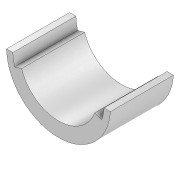
# Autodesk Inventor part: Back cover of tilting head
Saved by Autodesk Inventor 2020.3 (Build 243373010, 373A)
## iProperties
Created: 2021-05-15
Part Number: Back cover of tilting head
Material: Stainless Steel, Austenitic
Document SubType Name: Modeling
Designer: marti
Density: 8 g/cm^3
Appearance: Semi-Polished
Author: marti
Autodesk Inventor part; units mm, degrees
ref_plane "YZ Plane" through (0, 0, 0) normal (1, 0, 0) x (0, 1, 0)
ref_plane "XZ Plane" through (0, 0, 0) normal (0, 1, 0) x (-1, 0, 0)
ref_plane "XY Plane" through (0, 0, 0) normal (0, 0, 1) x (1, 0, 0)
sketch "Sketch1" plane through (0, 0, 0) normal (0, 0, 1) x (1, 0, 0)
  arc A0 (-41.2079, -77.8519) -> (41.1837, -79.7905) centre (0.0321, -76.9422) ccw
  line L0 (41.1837, -79.7905) -> (36.1791, -79.6728)
  arc A1 (34.3384, -88.653) -> (36.1791, -79.6728) centre (0.0321, -76.9422) ccw
  arc A2 (-36.2065, -77.8519) -> (-34.787, -87.0265) centre (0.0321, -76.9422) ccw
  line L1 (-29.2781, -85.431) -> (-34.787, -87.0265)
  line L2 (34.3384, -88.653) -> (28.8148, -86.7675)
  line L3 (-36.2065, -77.8519) -> (-41.2079, -77.8519)
  arc A3 (-30.7072, -77.6538) -> (-30.6804, -78.0996) centre (0, -76.0312) ccw
  arc A4 (-29.2781, -85.431) -> (28.8148, -86.7675) centre (0, -76.0312) ccw
  point P0 (0, 0)
  constraints: 10 point on circle, 8 end point, 5 centre point, 1 horizontal, 1 point on line
extrude "Extrusion1" add sketch "Sketch1" along normal mid plane 50
body "Solid1"
